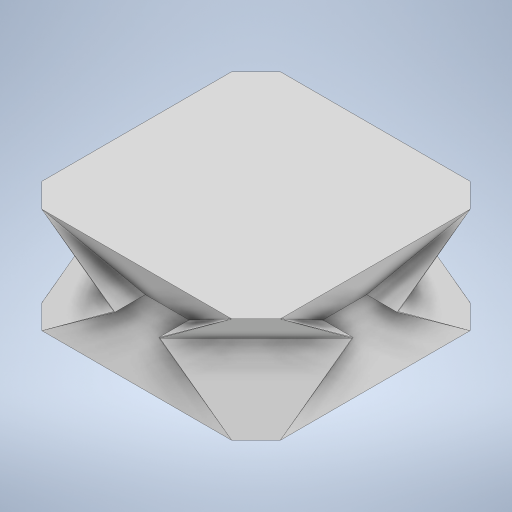
# Autodesk Inventor part: OV-PAM_NEW_SHAPE_5_patterns_1f_46_부피 구하기
Saved by Autodesk Inventor 2024 (Build 280153000, 153)
## iProperties
Created: 2023-06-26
Part Number: OV-PAM_NEW_SHAPE_5_patterns_1f_46_부피 구하기
Material: 일반
Document SubType Name: Modeling
Designer: jsw
Density: 1 g/cm^3
Appearance: 기본값
Mass: 53.8866 g
Surface Area: 125.084 cm^2
Volume: 53.8866 cm^3
Author: jsw
Autodesk Inventor part; units mm, degrees
ref_plane "YZ Plane" through (0, 0, 0) normal (1, 0, 0) x (0, 1, 0)
sketch "스케치1" plane through (0, 0, 0) normal (0, 1, 0) x (-1, 0, 0)
  line L0 (27.2, -11.2666) -> (11.2666, -27.2)
  line L1 (11.2666, -27.2) -> (-11.2666, -27.2)
  line L2 (-11.2666, -27.2) -> (-27.2, -11.2666)
  line L3 (-27.2, -11.2666) -> (-27.2, 11.2666)
  line L4 (-27.2, 11.2666) -> (-11.2666, 27.2)
  line L5 (-11.2666, 27.2) -> (11.2666, 27.2)
  line L6 (11.2666, 27.2) -> (27.2, 11.2666)
  line L7 (27.2, 11.2666) -> (27.2, -11.2666)
  line L8 (27.2, 11.2666) -> (27.2, 21.6686)
  line L9 (11.2666, 27.2) -> (21.6686, 27.2)
  line L10 (21.6686, 27.2) -> (27.2, 21.6686)
  line L11 (-11.2666, 27.2) -> (-21.6686, 27.2)
  line L12 (-27.2, 21.6686) -> (-21.6686, 27.2)
  line L13 (-27.2, 11.2666) -> (-27.2, 21.6686)
  line L14 (-27.2, -11.2666) -> (-27.2, -21.6686)
  line L15 (-21.6686, -27.2) -> (-27.2, -21.6686)
  line L16 (-11.2666, -27.2) -> (-21.6686, -27.2)
  line L17 (11.2666, -27.2) -> (21.6686, -27.2)
  line L18 (27.2, -21.6686) -> (21.6686, -27.2)
  line L19 (27.2, -11.2666) -> (27.2, -21.6686)
  line L20 (28, -11.598) -> (11.598, -28)
  line L21 (11.598, -28) -> (-11.598, -28)
  line L22 (-11.598, -28) -> (-28, -11.598)
  line L23 (-28, -11.598) -> (-28, 11.598)
  line L24 (-28, 11.598) -> (-11.598, 28)
  line L25 (-11.598, 28) -> (11.598, 28)
  line L26 (11.598, 28) -> (28, 11.598)
  line L27 (28, 11.598) -> (28, -11.598)
  line L28 (28, 11.598) -> (28, 22)
  line L29 (11.598, 28) -> (22, 28)
  line L30 (22, 28) -> (28, 22)
  line L31 (-11.598, 28) -> (-22, 28)
  line L32 (-28, 22) -> (-22, 28)
  line L33 (-28, 11.598) -> (-28, 22)
  line L34 (-28, -11.598) -> (-28, -22)
  line L35 (-22, -28) -> (-28, -22)
  line L36 (-11.598, -28) -> (-22, -28)
  line L37 (11.598, -28) -> (22, -28)
  line L38 (28, -22) -> (22, -28)
  line L39 (28, -11.598) -> (28, -22)
  point P0 (0, 0)
  point P1 (0, 0)
  point P2 (0, 0)
  point P3 (27.2, -11.2666)
  point P4 (24.4343, 24.4343)
  point P5 (-24.4343, -24.4343)
  point P6 (0, 0)
  point P7 (0, 0)
  point P8 (0, 0)
  point P9 (25, 25)
  point P10 (-25, -25)
  dimension "d7" = 360
  dimension "d35" = 360
  dimension "d38" = 50
  dimension "d39" = 56
  dimension "d40" = 0.8
  dimension "d41" = 0.8
  constraints: 80 end point, 5 coincident, 4 horizontal, 4 midpoint, 2 perpendicular, 2 vertical, 92 other
  measures "d38" horizontal distance of point (25, 25) point (-25, -25)
  measures "d39" distance between parallel lines of L25 L21
  measures "d40" distance between parallel lines of L38 L18
  measures "d41" distance between parallel lines of L27 L7
extrude "돌출1" add sketch "스케치1" along normal blind 12 contours L19 L20 L17 L0 | L0 L1 L2 L3 L4 L5 L6 L7 | L6 L9 L26 L8 | L19 L18 L17 L20 | L16 L22 L14 L2 | L26 L9 L10 L8 | L16 L15 L14 L22 | L4 L13 L24 L11 | L24 L13 L12 L11
ref_plane "작업 평면3" through (21.6686, 0, -27.2) normal (0, -0.5, 0.8660254) x (-1, 0, 0)
ref_plane "작업 평면4" through (27.2, 0, -21.6686) normal (-0.5086501, -0.6946584, 0.5086501) x (-0.7071068, 0, -0.7071068)
sketch "스케치4" plane through (21.6686, 0, -27.2) normal (0, 0, -1) x (-1, 0, 0)
  line L0 (0, 0) -> (43.3373, 0) projected
  line L1 (0, 0) -> (16.6686, 12)
  line L2 (0, 12) -> (43.3373, 12) projected
  line L3 (48.8686, 0) -> (43.3373, 0) projected
  line L4 (43.3373, 0) -> (26.6686, 12)
  point P0 (21.6686, 0)
  point P1 (21.6686, 12)
  dimension "d15" = 5
  dimension "d16" = 10
  constraints: 4 end point, 1 midpoint, 1 point on line
  measures "d15" distance of L1.end point (21.669, 12)
  measures "d16" distance of L1.end L4.end
extrude "돌출2" cut sketch "스케치4" against normal up to surface surface through (21.6686, 0, -27.2) normal (0, -0.5, 0.8660254)
sketch "스케치5" plane through (27.2, 0, -21.6686) normal (0.7071068, 0, -0.7071068) x (-0.7071068, 0, -0.7071068)
  line L0 (7.8225, 0) -> (0, 0) projected
  line L1 (0, 0) -> (-20.7846, 12)
  line L2 (0, 12) -> (-30.6441, 12) projected
  line L3 (38.4666, 0) -> (7.8225, 0) projected
  line L4 (7.8225, 0) -> (28.6071, 12)
  line L5 (38.4666, 12) -> (7.8225, 12) projected
  line L6 (-20.7846, 12) -> (28.6071, 12)
  line L7 (7.8225, 0) -> (0, 0)
  point P0 (3.9113, 0)
  point P1 (7.8225, 12)
  point P2 (0, 12)
  dimension "d19" = 150
  dimension "d20" = 150
  constraints: 8 end point, 2 collinear, 2 point on line
  measures "d19" angle of L4 L0
  measures "d20" angle of L1 L0
extrude "돌출3" cut sketch "스케치5" against normal up to surface surface through (27.2, 0, -21.6686) normal (-0.5086501, -0.6946584, 0.5086501)
pattern_circular "원형 패턴1" count 4 over 360 about axis through (0, -10, 0) along (0, 1, 0) of "돌출2", "돌출3"
mirror "미러2" about plane through (0, 12, 0) normal (0, 1, 0) of "돌출2", "돌출3", "원형 패턴1", "돌출1"
equation "\"d15\" = 0.5 * d16"
